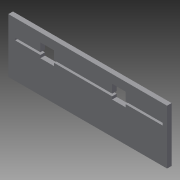
# Autodesk Inventor part: FrontBulkhead
Saved by Autodesk Inventor 2014 (Build 180170000, 170)
## iProperties
Created: 2015-01-07
Part Number: FrontBulkhead
Material: Generic
Document SubType Name: Modeling
Designer: Owner
Density: 1 g/cm^3
Appearance: Default
Author: Owner
Autodesk Inventor part; units mm, degrees
ref_plane "YZ Plane" through (0, 0, 0) normal (1, 0, 0) x (0, 1, 0)
ref_plane "XZ Plane" through (0, 0, 0) normal (0, 1, 0) x (-1, 0, 0)
ref_plane "XY Plane" through (0, 0, 0) normal (0, 0, 1) x (1, 0, 0)
sketch "Sketch1" plane through (0, 0, 0) normal (0, 0, 1) x (1, 0, 0)
  line L0 (117.4905, 295.341) -> (6.3655, 295.341)
  line L1 (6.3655, 295.341) -> (6.3655, 257.241)
  line L2 (6.3655, 257.241) -> (117.4905, 257.241)
  line L3 (117.4905, 257.241) -> (117.4905, 295.341)
  line L4 (117.4905, 283.403) -> (6.3655, 283.403)
  line L5 (6.3655, 283.403) -> (6.3655, 281.773)
  line L6 (6.3655, 281.773) -> (117.4905, 281.773)
  line L7 (117.4905, 281.773) -> (117.4905, 283.403)
  line L8 (117.4905, 281.773) -> (117.4905, 283.403)
  line L9 (6.3655, 283.403) -> (11.128, 283.403)
  line L10 (11.128, 283.403) -> (11.128, 281.773)
  line L11 (11.128, 281.773) -> (6.3655, 281.773)
  line L12 (6.3655, 281.773) -> (6.3655, 283.403)
  line L13 (117.4905, 283.403) -> (114.3155, 283.403)
  line L14 (114.3155, 283.403) -> (114.3155, 281.773)
  line L15 (114.3155, 281.773) -> (117.4905, 281.773)
  line L16 (117.4905, 281.773) -> (117.4905, 283.403)
  point P0 (0, 0)
  dimension "d0" = 38.1
  dimension "d1" = 111.125
  dimension "d2" = 1.63
  dimension "d3" = 11.938
  dimension "d23" = 103.1875
  dimension "d24" = 3.175
  constraints: 34 end point, 8 parallel, 6 point on line, 5 perpendicular, 4 horizontal
  measures "d0" distance of L0.end L1.end
  measures "d1" distance of L0.start L0.end
  measures "d2" distance between parallel lines of L6 L4
  measures "d3" distance between parallel lines of L0 L4
  measures "d23" distance between parallel lines of L14 L10
  measures "d24" distance between parallel lines of L3 L14
extrude "Extrusion1" add sketch "Sketch1" along normal blind 3.175 contours L3 L4 L1 L0 | L3 L6 L14 L4 | L4 L10 L6 L1 | L3 L2 L1 L6
sketch "Sketch2" plane through (0, 0, 0) normal (0, 0, -1) x (-1, 0, 0)
  line L0 (-114.3155, 283.403) -> (-11.128, 283.403) projected
  line L1 (-38.3069, 289.3188) -> (-28.7819, 289.3188)
  line L2 (-28.7819, 289.3188) -> (-28.7819, 279.7938)
  line L3 (-28.7819, 279.7938) -> (-38.3069, 279.7938)
  line L4 (-38.3069, 279.7938) -> (-38.3069, 289.3188)
  line L5 (-88.5327, 289.3772) -> (-79.0077, 289.3772)
  line L6 (-79.0077, 289.3772) -> (-79.0077, 279.8594)
  line L7 (-79.0077, 279.8594) -> (-88.5327, 279.8594)
  line L8 (-88.5327, 279.8594) -> (-88.5327, 289.3772)
  line L9 (-6.3655, 257.241) -> (-117.4905, 257.241) projected
  line L10 (-67.3255, 257.241) -> (-44.4655, 257.241)
  line L11 (-117.4905, 295.341) -> (-6.3655, 295.341) projected
  line L12 (-53.9905, 295.341) -> (-41.2905, 295.341)
  point P0 (0, 0)
  point P1 (-117.4905, 283.403)
  point P2 (-6.3655, 283.403)
  dimension "d8" = 9.525
  dimension "d9" = 9.5177
  dimension "d10" = 9.525
  dimension "d11" = 9.525
  dimension "d13" = 5.9159
  constraints: 20 end point, 4 horizontal, 4 parallel, 2 perpendicular, 2 point on line
  measures "d8" distance of L5.start L5.end
  measures "d9" distance of L5.end L6.end
  measures "d10" distance of L1.start L1.end
  measures "d11" distance of L3.end L1.start
  measures "d13" distance between parallel lines of L0 L1
extrude "Extrusion2" cut sketch "Sketch2" against normal blind 3.175
body "Solid1"
